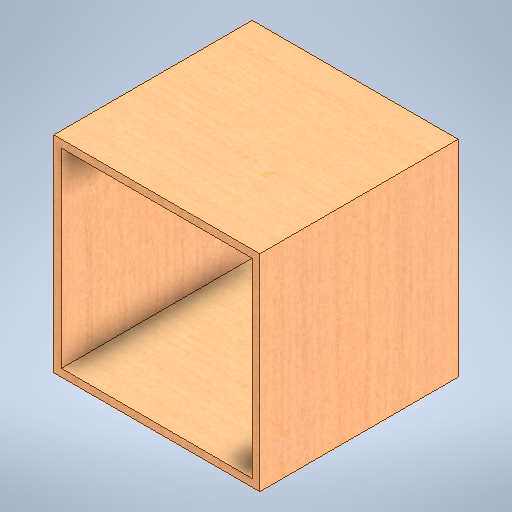
# Autodesk Inventor part: Estacion
Saved by Autodesk Inventor 2025.2 (Build 292293000, 293)
## iProperties
Created: 2025-05-21
Part Number: Estacion
Material: Wood (Cherry)
Document SubType Name: Modeling
Designer: USER
Density: 0.63 g/cm^3
Appearance: Cherry - Natural Low Gloss
Author: USER
Autodesk Inventor part; units mm, degrees
ref_plane "YZ Plane" through (0, 0, 0) normal (1, 0, 0) x (0, 1, 0)
ref_plane "XZ Plane" through (0, 0, 0) normal (0, 1, 0) x (-1, 0, 0)
ref_plane "XY Plane" through (0, 0, 0) normal (0, 0, 1) x (1, 0, 0)
sketch "Sketch1" plane through (0, 0, 0) normal (0, 1, 0) x (-1, 0, 0)
  line L0 (0, 0) -> (162, 0)
  line L1 (162, 0) -> (162, -156)
  line L2 (162, -156) -> (0, -156)
  line L3 (0, -156) -> (0, 0)
  dimension "d0" = 162
  dimension "d1" = 156
  constraints: 8 end point, 2 parallel, 1 horizontal, 1 perpendicular
  measures "d0" distance of L1.end L2.end
  measures "d1" distance of L0.end L1.end
extrude "Extrusion1" add sketch "Sketch1" along normal blind 6
sketch "Sketch3" plane through (0, 0, 0) normal (1, 0, 0) x (0, 0, -1)
  line L0 (156, 6) -> (0, 6) projected
  line L1 (0, 6) -> (156, 6)
  line L2 (156, 6) -> (156, 156)
  line L3 (156, 156) -> (0, 156)
  line L4 (0, 156) -> (0, 6)
  point P0 (0, 0)
  dimension "d4" = 150
  constraints: 8 end point, 2 parallel, 1 horizontal, 1 perpendicular
  measures "d4" distance of L2.end L1.end
extrude "Extrusion2" add sketch "Sketch3" against normal blind 6
sketch "Sketch4" plane through (-162, 0, -156) normal (-1, 0, 0) x (0, 0, 1)
  line L0 (0, 6) -> (156, 6) projected
  line L1 (156, 156) -> (0, 156) projected
  line L2 (0, 6) -> (156, 6)
  line L3 (156, 6) -> (156, 156)
  line L4 (156, 156) -> (0, 156)
  line L5 (0, 156) -> (0, 6)
  point P0 (156, 0)
  constraints: 8 end point, 2 parallel, 1 horizontal, 1 perpendicular
extrude "Extrusion3" add sketch "Sketch4" against normal blind 6
sketch "Sketch5" plane through (-162, 156, 0) normal (0, 1, 0) x (1, 0, 0)
  line L0 (0, 156) -> (0, 0) projected
  line L1 (162, 156) -> (0, 156)
  line L2 (0, 156) -> (0, 0)
  line L3 (0, 0) -> (162, 0)
  line L4 (162, 0) -> (162, 156)
  point P0 (162, 0)
  constraints: 8 end point, 2 parallel, 1 horizontal, 1 perpendicular
extrude "Extrusion4" add sketch "Sketch5" along normal blind 6
body "Solid1"
